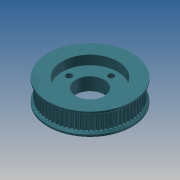
# Autodesk Inventor part: screw pulley
Saved by Autodesk Inventor 2013 (Build 170138000, 138)
## iProperties
Created: 2017-04-04
Part Number: screw pulley
Material: Generic
Document SubType Name: Modeling
Designer: employee
Density: 1 g/cm^3
Author: employee
Autodesk Inventor part; units mm, degrees
ref_plane "YZ Plane" through (0, 0, 0) normal (1, 0, 0) x (0, 1, 0)
ref_plane "XZ Plane" through (0, 0, 0) normal (0, 1, 0) x (-1, 0, 0)
ref_plane "XY Plane" through (0, 0, 0) normal (0, 0, 1) x (1, 0, 0)
sketch "Sketch1" plane through (0, 0, 0) normal (0, 0, 1) x (1, 0, 0)
  circle A0 centre (0, 0) radius 22.2817
  dimension "d0" = 44.5634
  constraints: 1 centre point, 1 coincident
  measures "d0" diameter of A0
extrude "Extrusion1" add sketch "Sketch1" along normal mid plane 8
sketch "Sketch3" plane through (0, 0, 4) normal (0, 0, 1) x (1, 0, 0)
  circle A0 centre (0, 0) radius 22.2817 projected
  circle A1 centre (0, 0) radius 22.0277
  dimension "d22" = 0.254
  constraints: 1 centre point
  measures "d22" radial gap between concentric circles of A0 A1
extrude "Extrusion3" cut sketch "Sketch3" against normal through all
sketch "Sketch4" plane through (0, 0, 4) normal (0, 0, 1) x (1, 0, 0)
  circle A0 centre (0, 0) radius 22.0277 projected
  circle A1 centre (0, 22.0277) radius 0.795
  dimension "d25" = 1.59
  constraints: 2 vertical alignment, 1 centre point, 1 other
  measures "d25" diameter of A1
extrude "Extrusion4" cut sketch "Sketch4" against normal through all contours A1 A0 | A0 A1 picked at (0.0316, 21.7635) picked at (0.0298, 22.29)
pattern_circular "Circular Pattern1" count 70 over 360 about axis through (0, 0, 4) along (0, 0, -1) of "Extrusion4"
sketch "Sketch5" plane through (0, 0, 4) normal (0, 0, 1) x (1, 0, 0)
  arc A0 (-19.7615, 9.7315) -> (-19.9295, 9.3827) centre (0, 0) ccw projected
  arc A1 (-0.7949, 22.0133) -> (-1.1816, 21.996) centre (0, 0) ccw projected
  circle A2 centre (0, 0) radius 23.0277
  dimension "d33" = 1
  constraints: 1 centre point, 1 coincident
  measures "d33" radial gap between concentric circles of A2 A0
extrude "Extrusion5" add sketch "Sketch5" along normal blind 2
chamfer "Chamfer1" distance 1 angle 45 1 edges at (-23.0277, 0, 4)
mirror "Mirror1" about plane through (0, 0, 0) normal (0, 0, 1) of "Extrusion5", "Chamfer1"
sketch "Sketch6" plane through (0, 0, 6) normal (0, 0, 1) x (1, 0, 0)
  circle A0 centre (0, 0) radius 23.0277 projected
  circle A1 centre (0, 0) radius 7.75
  dimension "d39" = 15.5
  constraints: 1 centre point, 1 coincident
  measures "d39" diameter of A1
extrude "Extrusion6" cut sketch "Sketch6" against normal through all contours A1
sketch "Sketch8" plane through (0, 0, 6) normal (0, 0, 1) x (1, 0, 0)
  circle A0 centre (0, 0) radius 7.75 projected
  circle A1 centre (0, 0) radius 23.0277 projected
  circle A2 centre (0, 0) radius 15.25
  dimension "d46" = 30.5
  constraints: 1 centre point, 1 coincident
  measures "d46" diameter of A2
extrude "Extrusion8" cut sketch "Sketch8" against normal blind 5 contours A2
sketch "Sketch9" plane through (0, 0, 1) normal (0, 0, 1) x (1, 0, 0)
  circle A0 centre (0, 0) radius 7.75 projected
  circle A1 centre (0, 11.5) radius 1.65
  dimension "d50" = 3.3
  dimension "d52" = 11.5
  constraints: 1 centre point, 1 vertical alignment
  measures "d50" diameter of A1
  measures "d52" distance of A0.centre A1.centre
extrude "Extrusion9" cut sketch "Sketch9" against normal through all contours A1
pattern_circular "Circular Pattern2" count 4 over 360 about axis through (0, 0, 6) along (0, 0, -1) of "Extrusion9"
body "Solid1"
